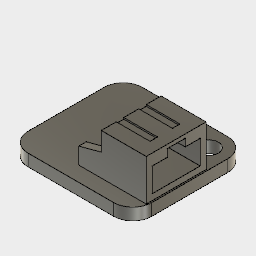
2124 Trinket Lipo Backpack (Autodesk Fusion 360 design; units mm, degrees)
Autodesk Fusion 360 part; units mm, degrees
sketch "Sketch1" plane through (0, 0, 0) normal (0, 0, 1) x (1, 0, 0)
  line L0 (0, 0) -> (16.51, 0)
  line L1 (16.51, 0) -> (16.51, 15.24)
  line L2 (16.51, 15.24) -> (0, 15.24)
  line L3 (0, 15.24) -> (0, 0)
  circle A0 centre (13.97, 12.7) radius 1.27
  dimension "d1" = 16.51
  dimension "d2" = 15.24
  dimension "d3" = 2.54
  dimension "d4" = 2.54
  dimension "d5" = 2.54
  measures "d1" distance of L0.start L0.end
  measures "d2" distance of L0.start L2.end
  measures "d3" diameter of A0
  measures "d4" distance of L2 A0.centre
  measures "d5" distance of L1 A0.centre
extrude "Extrude1" add sketch "Sketch1" against normal blind 1.6 makes body 1
fillet "Fillet1" radius 2.54 4 edges at (0, 15.24, -0.8) (16.51, 0, -0.8) (0, 0, -0.8) (16.51, 15.24, -0.8) on bodies 1
sketch "Sketch2" plane through (0, 0, 0) normal (0, 0, 1) x (-1, 0, 0)
  circle A0 centre (-13.97, -12.7) radius 1.27
  arc A1 (-16.51, -12.7) -> (-13.97, -15.24) centre (-13.97, -12.7) ccw
  line L0 (-13.97, -15.24) -> (-2.54, -15.24)
  arc A2 (-2.54, -15.24) -> (0, -12.7) centre (-2.54, -12.7) ccw
  line L1 (0, -12.7) -> (0, -2.54)
  arc A3 (0, -2.54) -> (-2.54, 0) centre (-2.54, -2.54) ccw
  line L2 (-2.54, 0) -> (-13.97, 0)
  arc A4 (-13.97, 0) -> (-16.51, -2.54) centre (-13.97, -2.54) ccw
  line L3 (-16.51, -2.54) -> (-16.51, -12.7)
  line L4 (-16.31, -10) -> (-10.31, -10)
  line L5 (-10.31, -10) -> (-10.31, -2)
  line L6 (-10.31, -2) -> (-16.31, -2)
  line L7 (-16.31, -2) -> (-16.31, -10)
  line L8 (-10.31, -10) -> (-7.31, -10)
  line L9 (-7.31, -10) -> (-7.31, -9)
  line L10 (-7.31, -9) -> (-10.31, -9)
  line L11 (-10.31, -9) -> (-10.31, -10)
  line L12 (-10.31, -2) -> (-7.31, -2)
  line L13 (-7.31, -2) -> (-7.31, -3)
  line L14 (-7.31, -3) -> (-10.31, -3)
  line L15 (-10.31, -3) -> (-10.31, -2)
  dimension "d9" = 8
  dimension "d10" = 6
  dimension "d11" = 0.2
  dimension "d13" = 2
  dimension "d16" = 3
  dimension "d17" = 1
  dimension "d18" = 3
  dimension "d19" = 1
  measures "d9" distance of L4.start L6.end
  measures "d10" distance of L5.end L6.end
  measures "d11" distance of L3 L7
  measures "d13" distance of L2 L6
  measures "d16" distance of L4.end L8.end
  measures "d17" distance of L4.end L10.end
  measures "d18" distance of L5.end L12.end
  measures "d19" distance of L5.end L14.end
extrude "Extrude2" add sketch "Sketch2" along normal blind 5.5 separate body contours L4 L5 L6 L7 L11 L15 makes body 2
extrude "Extrude3" add sketch "Sketch2" along normal blind 3 contours L5 L8 L9 L10 L11 | L5 L12 L13 L14 L15 bodies 1 2
draft "Draft1" angle 15 neutral plane through (10.31, 3, 0) pull (-1, 0, 0) 1 faces at (9.31, 9.3333, 3) on bodies 1
draft "Draft2" angle 15 neutral plane through (10.31, 3, 0) pull (-1, 0, 0) 1 faces at (8.31, 2.6667, 3) on bodies 1
sketch "Sketch3" plane through (0, 0, 5.5) normal (0, 0, 1) x (-1, 0, 0)
  line L0 (-16.31, -2) -> (-16.31, -10)
  line L1 (-16.31, -10) -> (-10.31, -10)
  line L2 (-10.31, -10) -> (-10.31, -2)
  line L3 (-10.31, -2) -> (-16.31, -2)
  line L4 (-10.31, -8) -> (-14.81, -8)
  line L5 (-14.81, -8) -> (-14.81, -7)
  line L6 (-14.81, -7) -> (-10.31, -7)
  line L7 (-10.31, -7) -> (-10.31, -8)
  line L8 (-16.31, -10) -> (-10.31, -10)
  line L9 (-10.31, -4) -> (-14.81, -4)
  line L10 (-14.81, -4) -> (-14.81, -5)
  line L11 (-14.81, -5) -> (-10.31, -5)
  line L12 (-10.31, -5) -> (-10.31, -4)
  line L13 (-10.31, -2) -> (-16.31, -2)
  dimension "d26" = 4.5
  dimension "d27" = 1
  dimension "d28" = 2
  dimension "d29" = 4.5
  dimension "d30" = 1
  dimension "d31" = 2
  measures "d26" distance of L4.start L4.end
  measures "d27" distance of L4.start L6.end
  measures "d28" distance of L4 L8
  measures "d29" distance of L9.start L9.end
  measures "d30" distance of L9.start L11.end
  measures "d31" distance of L9 L13
extrude "Extrude4" cut sketch "Sketch3" against normal blind 0.2 contours L2 L9 L10 L11 L12 | L2 L4 L5 L6 L7 bodies 1
sketch "Sketch4" plane through (16.31, 0, 0) normal (1, 0, 0) x (0, 1, 0)
  line L0 (2, 0) -> (10, 0)
  line L1 (10, 0) -> (10, 5.5)
  line L2 (10, 5.5) -> (2, 5.5)
  line L3 (2, 5.5) -> (2, 0)
  line L4 (2.8, 0.8) -> (9.2, 0.8)
  line L5 (9.2, 0.8) -> (9.2, 4)
  line L6 (9.2, 4) -> (7.2, 4)
  line L7 (7.2, 4) -> (7.2, 5)
  line L8 (7.2, 5) -> (4.8, 5)
  line L9 (4.8, 5) -> (4.8, 4)
  line L10 (4.8, 4) -> (2.8, 4)
  line L11 (2.8, 4) -> (2.8, 0.8)
  line L12 (6, 5.5) -> (6, 0) construction
  line L13 (2, 0) -> (10, 0)
  dimension "d34" = 0.8
  dimension "d35" = 0.8
  dimension "d36" = 0.8
  dimension "d37" = 1.2
  dimension "d38" = 1.2
  dimension "d39" = 1.5
  dimension "d40" = 1.5
  measures "d34" distance of L3 L11
  measures "d35" distance of L1 L5
  measures "d36" distance of L4 L13
  measures "d37" distance of L9 L12
  measures "d38" distance of L7 L12
  measures "d39" distance of L2 L6
  measures "d40" distance of L2 L10
extrude "Extrude5" cut sketch "Sketch4" against normal blind 5.2 contours L4 L5 L6 L7 L8 L9 L10 L11 bodies 1
